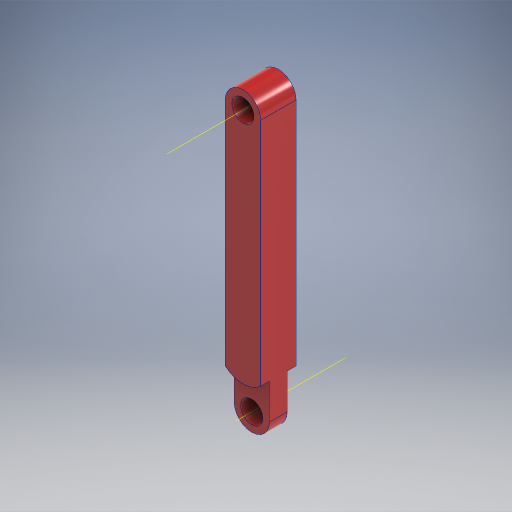
# Autodesk Inventor part: link7
Saved by Autodesk Inventor 2024.1 (Build 281209000, 209)
## iProperties
Created: 2023-09-09
Part Number: link7
Material: Aluminum 6061
Document SubType Name: Modeling
Designer: Camilo
Density: 2.7 g/cm^3
Appearance: Aluminum - Flat
Mass: 1.24114 g
Surface Area: 6.06202 cm^2
Volume: 0.45968 cm^3
Author: Camilo
Autodesk Inventor part; units mm, degrees
ref_plane "YZ Plane" through (0, 0, 0) normal (1, 0, 0) x (0, 1, 0)
ref_plane "XZ Plane" through (0, 0, 0) normal (0, 1, 0) x (-1, 0, 0)
ref_plane "XY Plane" through (0, 0, 0) normal (0, 0, 1) x (1, 0, 0)
sketch "Sketch6" plane through (0, 0, 0) normal (0, 0, 1) x (1, 0, 0)
  line L0 (0, 0) -> (0, 15)
  line L1 (0, 15) -> (2, 15)
  line L2 (2, 15) -> (-2, 15)
  line L3 (-2, 15) -> (-2, -15)
  line L4 (-2, -15) -> (2, -15)
  line L5 (2, -15) -> (2, 15)
  circle A0 centre (0, 15) radius 1.25
  circle A1 centre (0, 15) radius 2
  circle A2 centre (0, -15) radius 1.25
  circle A3 centre (0, -15) radius 2
  line L6 (-2, -15) -> (-2, -11)
  line L7 (2, -15) -> (2, -11)
  line L8 (-2, 15) -> (2, 15)
  line L9 (2, 15) -> (2, 14)
  line L10 (2, 14) -> (-2, 14)
  line L11 (-2, 14) -> (-2, 15)
  arc A4 (-2, 14) -> (2, 14) centre (0, 14) ccw
  arc A5 (-2, -11) -> (2, -11) centre (0, -8.7639) ccw
  point P0 (-2, 14)
  point P1 (0, 12)
  point P2 (0, 13.75)
  point P3 (1.25, 15)
  dimension "d115" = 15
  dimension "d116" = 2
  dimension "d117" = 4
  dimension "d118" = 30
  dimension "d119" = 2.5
  dimension "d120" = 2.5
  dimension "d121" = 4
  dimension "d122" = 4
  dimension "d124" = 1
  dimension "d125" = 2
  dimension "d132" = 3
  constraints: 24 end point, 6 point on circle, 5 centre point, 4 parallel, 3 coincident, 3 perpendicular, 3 point on line, 2 horizontal, 1 midpoint, 1 vertical, 3 other
  measures "d115" distance of L0.start L0.end
  measures "d116" distance of L0.end L1.end
  measures "d117" distance of L4.end L3.end
  measures "d118" distance of L3.end L2.end
  measures "d119" diameter of A0
  measures "d120" diameter of A2
  measures "d121" distance of L6.start L6.end
  measures "d122" distance of L4.end L7.end
  measures "d124" distance of L8.end L9.end
  measures "d125" radius of A4
  measures "d132" radius of A5
extrude "Extrusion8" add sketch "Sketch6" along normal mid plane 4 contours A4 L10 A1 L0 | A4 L5 A5 L3 | L0 A1 L10 A4 | A1 L10 A0 L0 | L0 A0 L10 A1 | L3 A1 L10 | L10 A1 L5 | A1 L2 A0 L10 | L10 A0 L1 A1 | A1 L1 A0 L2
extrude "Extrusion9" cut sketch "Sketch6" along normal mid plane 2 contours A3 L4 A2 | L4 A2 A3
extrude "Extrusion10" add sketch "Sketch6" along normal mid plane 2 contours A5 L5 A3 L3 | A3 L4 A2 | L4 A2 A3
body "Solid3"
